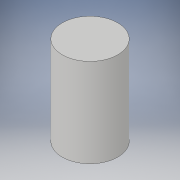
# Autodesk Inventor part: cslegs
Saved by Autodesk Inventor 2019 (Build 230136000, 136)
## iProperties
Created: 2020-02-18
Part Number: cslegs
Material: Generic
Document SubType Name: Modeling
Designer: Dell
Density: 1 g/cm^3
Appearance: Default
Author: Dell
Autodesk Inventor part; units mm, degrees
ref_plane "YZ Plane" through (0, 0, 0) normal (1, 0, 0) x (0, 1, 0)
ref_plane "XZ Plane" through (0, 0, 0) normal (0, 1, 0) x (-1, 0, 0)
ref_plane "XY Plane" through (0, 0, 0) normal (0, 0, 1) x (1, 0, 0)
sketch "Sketch1" plane through (0, 0, 0) normal (0, 1, 0) x (-1, 0, 0)
  circle A0 centre (0, 0) radius 25
  circle A1 centre (-16.1397, -19.0921) radius 0.2511
  dimension "d0" = 50
  constraints: 1 centre point, 1 coincident, 3 other
extrude "Extrusion1" add sketch "Sketch1" along normal blind 80 contours A0 A1 | A1 A0 picked at (5.9147, 5.8478) picked at (-16.0926, -19.0228)
body "Solid1"
